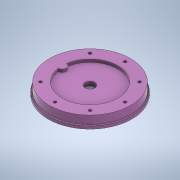
# Autodesk Inventor part: основание
Saved by Autodesk Inventor 2022 (Build 260153000, 153)
## iProperties
Created: 2024-04-28
Part Number: основание
Material: Типовые
Document SubType Name: Modeling
Designer: Pavel
Density: 1 g/cm^3
Appearance: По умолчанию
Mass: 2.33987 g
Surface Area: 20.2599 cm^2
Volume: 2.33987 cm^3
Author: Pavel
Autodesk Inventor part; units mm, degrees
ref_plane "YZ Plane" through (0, 0, 0) normal (1, 0, 0) x (0, 1, 0)
ref_plane "XZ Plane" through (0, 0, 0) normal (0, 1, 0) x (-1, 0, 0)
sketch "Эскиз2" plane through (0, 0, 0) normal (1, 0, 0) x (0, 1, 0)
  line L0 (0, 1.75) -> (2, 1.75)
  line L1 (2, 1.75) -> (2, 10)
  line L2 (2, 10) -> (3, 10)
  line L3 (3, 10) -> (3, 14.5)
  line L4 (3, 14.5) -> (0, 14.5)
  line L5 (0, 14.5) -> (0, 15)
  line L6 (0, 15) -> (-1, 15)
  line L7 (-1, 15) -> (-1, 5)
  line L8 (-1, 5) -> (-2, 5)
  line L9 (-2, 5) -> (-2, 0)
  line L10 (-2, 0) -> (0, 0)
  line L11 (0, 0) -> (0, 1.75)
  line L12 (-3, 0) -> (4, 0) projected
  dimension "d2" = 1.75
  dimension "d3" = 2
  dimension "d4" = 8.25
  dimension "d5" = 1
  dimension "d6" = 4.5
  dimension "d7" = 3
  dimension "d9" = 0.5
  dimension "d10" = 1
  dimension "d11" = 10
  dimension "d12" = 1
  constraints: 24 end point, 7 perpendicular, 1 parallel, 1 vertical
  measures "d2" distance of L10.end L0.start
  measures "d3" distance of L0.start L0.end
  measures "d4" distance of L0.end L1.end
  measures "d5" distance of L1.end L2.end
  measures "d6" distance of L2.end L3.end
  measures "d7" distance of L3.end L4.end
  measures "d9" distance of L4.end L5.end
  measures "d10" distance of L5.end L6.end
  measures "d11" distance of L6.end L7.end
  measures "d12" distance of L7.end L8.end
revolve "Вращение1" add sketch "Эскиз2" angle 360 about axis through (0, -10, 0) along (0, 1, 0)
sketch "Эскиз3" plane through (0, 3, 0) normal (0, 1, 0) x (1, 0, 0)
  circle A0 centre (0, 0) radius 10 projected
  circle A1 centre (-10, 0) radius 1.5
  point P0 (-9.8875, 1.4958)
  point P1 (-9.8875, -1.4958)
  dimension "d14" = 3
  constraints: 1 centre point, 2 other
  measures "d14" diameter of A1
extrude "Выдавливание1" add sketch "Эскиз3" against normal blind 1 contours A1 A0 picked at (-9.4917, 0)
ref_plane "РабПлоскость1" through (0, 1, 0) normal (0, 1, 0) x (1, 0, 0)
sketch "Эскиз5" plane through (0, 0, 0) normal (0, 0, 1) x (1, 0, 0)
  line L0 (14.5, 3) -> (-14.5, 3) construction
  line L1 (0, 3) -> (0, 1) construction
  line L2 (0, 1) -> (12.5, 1) construction
  circle A0 centre (12.5, 1) radius 1
  point P0 (0, 0)
  dimension "d20" = 2
  dimension "d21" = 12.5
  dimension "d22" = 2
  constraints: 4 end point, 1 centre point, 1 coincident, 1 midpoint, 1 perpendicular, 1 vertical
  measures "d20" distance of L1.start L1.end
  measures "d21" distance of L1.end L2.end
  measures "d22" diameter of A0
extrude "Выдавливание2" cut sketch "Эскиз5" along normal mid plane 0.5
sketch "Эскиз6" plane through (0, 3, 0) normal (0, 1, 0) x (1, 0, 0)
  circle A0 centre (0, 0) radius 12.5 construction
  circle A1 centre (12.5, 0) radius 0.5
  dimension "d25" = 25
  dimension "d26" = 1
  constraints: 1 centre point, 1 coincident, 1 horizontal alignment, 2 other
  measures "d26" diameter of A1
extrude "Выдавливание3" cut sketch "Эскиз6" against normal up to surface round surface about axis through (12.5, 1, 0) along (0, 0, 1) radius 1 far side no
sketch "Эскиз7" plane through (0, -1, 0) normal (0, -1, 0) x (1, 0, 0)
  circle A0 centre (12.5, 0) radius 0.5 projected
  circle A1 centre (12.5, 0) radius 0.5
  point P0 (0, 0)
  constraints: 1 centre point, 1 coincident
extrude "Выдавливание4" cut sketch "Эскиз7" against normal up to surface round surface about axis through (12.5, 1, 0) along (0, 0, 1) radius 1 far side no
pattern_circular "Круговой массив2" count 4 over 135 about axis through (0, 1, 0) along (0, 1, 0) of "Выдавливание4", "Выдавливание2", "Выдавливание3"
pattern_circular "Круговой массив3" count 4 over 135 about axis through (0, 1, 0) along (0, -1, 0) of "Выдавливание3", "Выдавливание2", "Выдавливание4"
sketch "Эскиз8" plane through (0, 0, 0) normal (0, 1, 0) x (1, 0, 0)
  circle A0 centre (0, 0) radius 1.75 projected
extrude "Выдавливание5" cut sketch "Эскиз8" against normal blind 10
sketch "Эскиз9" plane through (0, -2, 0) normal (0, -1, 0) x (1, 0, 0)
  circle A0 centre (0, 0) radius 3.5 construction
  circle A1 centre (0, 0) radius 1.75 projected
  line L0 (-3.5, 0) -> (-1.75, 3.0311)
  line L1 (-1.75, 3.0311) -> (1.75, 3.0311)
  line L2 (1.75, 3.0311) -> (3.5, 0)
  line L3 (3.5, 0) -> (1.75, -3.0311)
  line L4 (1.75, -3.0311) -> (-1.75, -3.0311)
  line L5 (-1.75, -3.0311) -> (-3.5, 0)
  dimension "d45" = 7
  constraints: 12 end point, 2 coincident, 1 horizontal alignment, 15 other
extrude "Выдавливание6" cut sketch "Эскиз9" against normal blind 2.5
